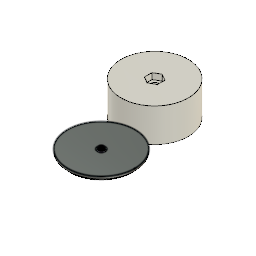
Project3D (Autodesk Fusion 360 design; units mm, degrees)
Autodesk Fusion 360 part; units mm, degrees
sketch "Cilindro" plane through (0, 0, 0) normal (0, 0, 1) x (1, 0, 0)
  circle A0 centre (0, 0) radius 30
  circle A1 centre (0, 0) radius 28
  circle A2 centre (0, 0) radius 3.475
  arc A3 (-5.1605, 1.9024) -> (-0.8047, -5.4408) centre (0, 0) ccw
  line L0 (0.75, -28.2428) -> (0.7433, -27.9901) construction
  line L1 (0.75, -28.2428) -> (0.7433, -27.9901) construction
  arc A4 (4.2277, 3.518) -> (-4.3095, 3.4173) centre (0, 0) ccw
  arc A5 (-5.1143, 2.0235) -> (-5.1605, 1.9024) centre (0, 0) ccw
  arc A6 (0.8047, -5.4408) -> (5.1143, 2.0235) centre (0, 0) ccw
  arc A7 (4.3095, 3.4173) -> (4.2277, 3.518) centre (0, 0) ccw
  line L2 (-0.0922, 3.4738) -> (-0.0922, 3.4738) construction
  line L3 (-0.0922, 3.4738) -> (0.0922, 3.4738) construction
  line L4 (0.8047, -5.4408) -> (0.8047, -27.9884)
  line L5 (-0.8047, -27.9884) -> (-0.8047, -5.4408)
  line L6 (0.0915, 3.4738) -> (0.1448, 5.4981) construction
  line L7 (4.3095, 3.4173) -> (23.8363, 14.6911)
  line L8 (24.6411, 13.2973) -> (5.1143, 2.0235)
  line L9 (-5.1143, 2.0235) -> (-24.6411, 13.2973)
  line L10 (-23.8363, 14.6911) -> (-4.3095, 3.4173)
  dimension "d9" = 56
  dimension "d10" = 6.95
  dimension "d11" = 11
  dimension "d113" = 60
  dimension "d116" = 360
  constraint concentric A1 A2
  constraint concentric A1 A6
  constraint coincident A0.centre A1.centre
  constraint concentric A3 A6
  constraint concentric A4 A6
  constraint coincident A3.start A5.end
  constraint coincident A4.start A7.end
  constraint coincident A0.centre L1
  constraint coincident A0.centre L0
  constraint coincident A2 L2.start
  constraint coincident A1 L0.end
  constraint concentric A4 A5
  constraint concentric A6 A7
  constraint collinear L2 L3
  constraint coincident A2 L3.end
  constraint coincident A4 L6.end
  constraint coincident L3 L6.start
  constraint coincident A1 L4.end
  constraint coincident A1 L5.start
  constraint parallel L4 L5
  measures "d9" diameter of A1
  measures "d10" diameter of A2
  measures "d11" diameter of A6
  measures "d113" diameter of A0
extrude "Extrude4" add sketch "Cilindro" against normal blind 2 contours A1 A6 L4 L8 | A1 A3 A4 A5 A6 A7 L4 L5 L7 L8 L9 L10 | A1 A4 A7 L7 L10 | A1 A3 A5 L5 L9 | A2 makes body 1
extrude "Extrude5" add sketch "Cilindro" against normal blind 30 contours A0 | A1 A3 A4 A5 A6 A7 L4 L5 L7 L8 L9 L10 bodies 1
extrude "Extrude6" cut 1 faces at (1.2629, 0.4165, -2) along direction (0, 0, 1) through all on bodies 1 bodies 1
copy_body "Body->Comp1" bodies 1 removing the originals makes body 2 in component "Cilindro"
sketch "Sketch17" plane through (0, 0, 0) normal (0, 0, 1) x (1, 0, 0)
  circle A0 centre (0, 0) radius 30
  circle A1 centre (0, 0) radius 27.7
  circle A2 centre (0, 0) radius 26
  circle A3 centre (0, 0) radius 2.975
  dimension "d102" = 60
  dimension "d105" = 55.4
  dimension "d106" = 52
  dimension "d111" = 5.95
  constraint coincident A0.centre A1.centre
  constraint concentric A0 A3
  measures "d102" diameter of A0
  measures "d105" diameter of A1
  measures "d106" diameter of A2
  measures "d111" diameter of A3
sketch "Sketch1" plane through (0, 0, 0) normal (0, 0, 1) x (-1, 0, 0) in component "Cilindro"
  circle A0 centre (0, 0) radius 3.475
  circle A1 centre (0, 0) radius 30
  circle A2 centre (0, 0) radius 8
  line L0 (-5.85, -3.3775) -> (0, -6.755)
  line L1 (0, -6.755) -> (5.85, -3.3775)
  line L2 (5.85, -3.3775) -> (5.85, 3.3775)
  line L3 (5.85, 3.3775) -> (0, 6.755)
  line L4 (0, 6.755) -> (-5.85, 3.3775)
  line L5 (-5.85, 3.3775) -> (-5.85, -3.3775)
  dimension "d119" = 16
  dimension "d122" = 5.85
  constraint coincident A0.centre A1.centre
  measures "d119" diameter of A2
  measures "d122" distance of A0.centre L5
extrude "Extrude6'" cut sketch "Sketch1" against normal blind 5.4 contours L0 L1 L2 L3 L4 L5 bodies 2 in component "Cilindro"
extrude "Extrude5'" add sketch "Sketch1" against normal blind 7 contours A2 | L0 L1 L2 L3 L4 L5 bodies 2 in component "Cilindro"
extrude "Extrude7" cut sketch "Sketch1" against normal blind 5.4 contours L0 L1 L2 L3 L4 L5 bodies 2 in component "Cilindro"
sketch "Sketch18" plane through (-32.7772, 56.7717, 0) normal (-0.5, 0.866025, 0) x (-0.866025, -0.5, 0)
  line L0 (-30.9733, 7.9112) -> (-33.4919, 7.9112)
  line L1 (-33.4919, 7.9112) -> (-33.4919, 12.9112)
  line L2 (-33.4919, 12.9112) -> (-53.5209, 12.9112)
  line L3 (-53.5209, 12.9112) -> (-53.5209, -15.0888)
  line L4 (-53.5209, -15.0888) -> (-30.9733, -15.0888)
  line L5 (-30.9733, -15.0888) -> (-30.9733, 7.9112)
  line L6 (-33.4663, 6.1337) -> (-4.4402, 6.3073) construction
  line L7 (-4.4402, 6.3073) -> (-4.4658, 10.5848) construction
  line L8 (-4.4658, 10.5848) -> (-33.4919, 10.4112) construction
  line L9 (-33.4919, 10.4112) -> (-33.4663, 6.1337) construction
  dimension "d127" = 3
  constraint midpoint L1
sketch "Sketch19" plane through (0, 0, -17.6649) normal (0, 0, -1) x (1, 0, 0)
  circle A0 centre (-23.7351, -67.226) radius 2.975
  circle A1 centre (-23.7351, -67.226) radius 30
sketch "Sketch20" plane through (0, 0, -21.9396) normal (0, 0, -1) x (1, 0, 0)
  line L0 (-21.8331, -64.9494) -> (-21.8331, -42.4018)
  arc A0 (2.0032, -83.6875) -> (-21.8331, -42.4018) centre (-22.6379, -70.3902) ccw
  line L1 (2.0032, -83.6875) -> (-17.5236, -72.4137)
  arc A1 (-17.5236, -72.4137) -> (-21.8331, -64.9494) centre (-22.6379, -70.3902) ccw
  line L2 (-18.3284, -73.8075) -> (1.1984, -85.0813)
  arc A2 (-46.4742, -85.0813) -> (1.1984, -85.0813) centre (-22.6379, -70.3902) ccw
  line L3 (-46.4742, -85.0813) -> (-26.9474, -73.8075)
  arc A3 (-26.9474, -73.8075) -> (-18.3284, -73.8075) centre (-22.6379, -70.3902) ccw
  circle A4 centre (-22.6379, -70.3902) radius 30
  arc A5 (-23.4426, -42.4018) -> (-47.2789, -83.6875) centre (-22.6379, -70.3902) ccw
  line L4 (-23.4426, -42.4018) -> (-23.4426, -64.9494)
  arc A6 (-23.4426, -64.9494) -> (-27.7521, -72.4137) centre (-22.6379, -70.3902) ccw
  line L5 (-27.7521, -72.4137) -> (-47.2789, -83.6875)
  circle A7 centre (-22.6379, -70.3902) radius 3.475
  circle A8 centre (-22.6379, -70.3902) radius 28
  constraint concentric A0 A8
extrude "Extrude8" cut sketch "Sketch20" against normal blind 2.5 contours L0 L1 A1 L2 L3 A3 L4 A6 L5 A8 sketch seen with x (1, 0, 0) y (0, 1, 0) z (0, 0, 1) at (22.6379, -70.3902, -8.0604) bodies 2 in component "Cilindro"
sketch "Sketch22" plane through (0, 0, 0) normal (0, 0, 1) x (1, 0, 0)
sketch "Sketch23" plane through (0, 0, 0) normal (0, 0, 1) x (1, 0, 0)
  circle A0 centre (0, 0) radius 30
  circle A1 centre (0, 0) radius 3.475
  dimension "d154" = 60
  dimension "d157" = 6.95
  constraint coincident A0.centre A1.centre
  constraint concentric A0 A1
  measures "d154" diameter of A0
  measures "d157" diameter of A1
extrude "Extrude1" add sketch "Sketch23" against normal blind 2 separate body makes body 3 in component "Component"
sketch "Sketch24" plane through (0, 0, -2) normal (0, 0, -1) x (1, 0, 0)
  circle A0 centre (0, 0) radius 3.475
  circle A1 centre (0, 0) radius 30
  circle A2 centre (0, 0) radius 27.7
  circle A3 centre (0, 0) radius 26
  dimension "d164" = 55.4
  dimension "d165" = 52
  constraint coincident A0.centre A1.centre
  constraint concentric A2 A3
  measures "d164" diameter of A2
  measures "d165" diameter of A3
extrude "Extrude2" add sketch "Sketch24" along normal blind 2.5 contours A2 bodies 3 in component "Component"
component "Cilindro" placed x (1, 0, 0) y (0, 1, 0) z (0, 0, 1) at (-22.6379, 70.3902, 8.0604)
component "Component" placed x (1, 0, 0) y (0, 1, 0) z (0, 0, 1) at (0, 0, 0)
